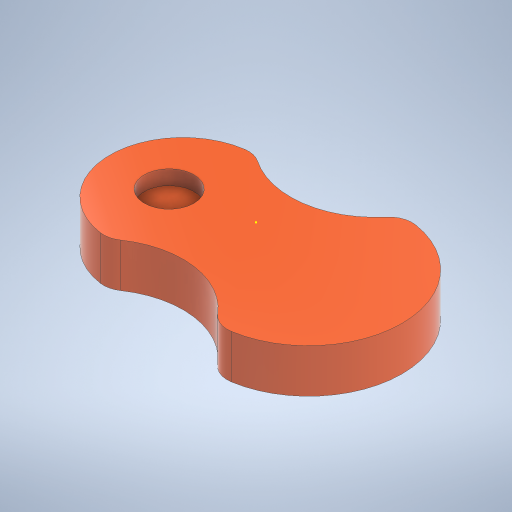
# Autodesk Inventor part: Axel
Saved by Autodesk Inventor 2024 (Build 280153020, 153B)
## iProperties
Created: 2023-09-12
Part Number: Axel
Material: Generic
Document SubType Name: Modeling
Designer: 23also
Density: 1 g/cm^3
Appearance: Default
Author: 23also
Autodesk Inventor part; units mm, degrees
ref_plane "YZ Plane" through (0, 0, 0) normal (1, 0, 0) x (0, 1, 0)
ref_plane "XZ Plane" through (0, 0, 0) normal (0, 1, 0) x (-1, 0, 0)
ref_plane "XY Plane" through (0, 0, 0) normal (0, 0, 1) x (1, 0, 0)
sketch "Sketch1" plane through (0, 0, 0) normal (0, 1, 0) x (-1, 0, 0)
  circle A0 centre (0, 0) radius 25
  dimension "d0" = 50
  constraints: 1 centre point, 1 coincident
  measures "d0" diameter of A0
extrude "Extrusion1" add sketch "Sketch1" along normal blind 10
sketch "Sketch2" plane through (0, 0, 0) normal (0, -1, 0) x (1, 0, 0)
  circle A0 centre (0, 0) radius 4.15
  dimension "d3" = 8.3
  constraints: 1 centre point, 1 coincident
  measures "d3" diameter of A0
extrude "Extrusion2" cut sketch "Sketch2" against normal blind 2.5
sketch "Sketch8" plane through (0, 10, 0) normal (0, 1, 0) x (1, 0, 0)
  point P0 (0, 0)
sketch "Sketch9" plane through (0, 10, 0) normal (0, 1, 0) x (1, 0, 0)
  circle A0 centre (0, 0) radius 25 projected
  circle A1 centre (-12.5, 0) radius 12.5
  circle A2 centre (9, 0) radius 16
  arc A3 (9, -16) -> (-12.5, -12.5) centre (-3.2934, -23.7306) ccw
  arc A4 (-12.5, 12.5) -> (9, 16) centre (-3.2934, 23.7306) ccw
  point P0 (-25, 0)
  point P1 (25, 0)
  dimension "d17" = 32
  constraints: 9 point on circle, 4 centre point
  measures "d17" diameter of A2
extrude "Extrusion6" cut sketch "Sketch9" against normal blind 15 contours A2 A1 A0 | A0 A1 A2 | A4 A2 | A2 A3 | A1 A4 | A3 A1
fillet "Fillet3" radius 4 1 edges at (-12.5, 5, 12.5)
fillet "Fillet4" radius 4 1 edges at (9, 5, 16)
fillet "Fillet5" radius 4 1 edges at (-12.5, 5, -12.5)
fillet "Fillet6" radius 4 1 edges at (9, 5, -16)
sketch "Sketch10" plane through (0, 10, 0) normal (0, 1, 0) x (1, 0, 0)
  circle A0 centre (0, 0) radius 4.15 projected
  circle A1 centre (0, 0) radius 29.3218
  constraints: 1 centre point, 1 coincident
extrude "Extrusion7" cut sketch "Sketch10" against normal blind 2.5 contours A0 | A1
sketch "Sketch11" plane through (0, 7.5, 0) normal (0, 1, 0) x (1, 0, 0)
  circle A0 centre (-14.875, 0) radius 4.25
  point P0 (0, 0)
  dimension "d26" = 8.5
  constraints: 1 centre point
  measures "d26" diameter of A0
extrude "Extrusion8" cut sketch "Sketch11" against normal blind 2.5
body "Solid1"
